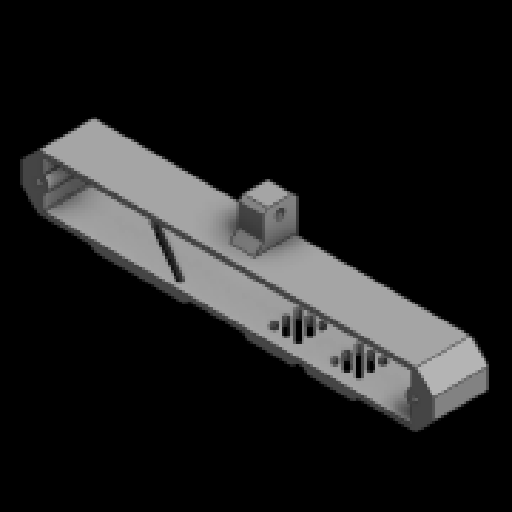
# Autodesk Inventor part: DepthCameraHousing
Saved by Autodesk Inventor 2025.2 (Build 292293000, 293)
## iProperties
Created: 2026-02-04
Part Number: DepthCameraHousing
Material: Generic
Document SubType Name: Modeling
Designer: valer
Density: 1 g/cm^3
Appearance: Default
Author: valer
Autodesk Inventor part; units mm, degrees
ref_plane "YZ Plane" through (0, 0, 0) normal (1, 0, 0) x (0, 1, 0)
ref_plane "XZ Plane" through (0, 0, 0) normal (0, 1, 0) x (-1, 0, 0)
ref_plane "XY Plane" through (0, 0, 0) normal (0, 0, 1) x (1, 0, 0)
sketch "Base" plane through (0, 0, 0) normal (0, 0, 1) x (1, 0, 0)
  line L0 (-81.75, 10.35) -> (81.75, 10.35)
  line L1 (81.75, 10.35) -> (81.75, -10.35)
  line L2 (81.75, -10.35) -> (-81.75, -10.35)
  line L3 (-81.75, -10.35) -> (-81.75, 10.35)
  line L4 (-81.75, 10.35) -> (81.75, -10.35) construction
  line L5 (81.75, 10.35) -> (-81.75, -10.35) construction
  line L6 (-122.5, 0) -> (122.5, 0) construction
  line L7 (0, -17.29) -> (0, 17.29) construction
  line L8 (83.75, 12.35) -> (-83.75, 12.35)
  line L9 (-83.75, 12.35) -> (-83.75, -12.35)
  line L10 (-83.75, -12.35) -> (83.75, -12.35)
  line L11 (83.75, -12.35) -> (83.75, 12.35)
  circle A0 centre (-83.5, 0) radius 4
  circle A1 centre (83.5, 0) radius 4
  line L12 (-83.5, 0) -> (83.5, 0) construction
  circle A2 centre (-83.5, 0) radius 1
  circle A3 centre (83.5, 0) radius 1
  point P0 (0, 0)
  point P1 (-83.75, 3.9922)
  point P2 (-83.75, -3.9922)
  point P3 (83.75, -3.9922)
  point P4 (83.75, 3.9922)
  point P5 (-81.75, 3.5969)
  point P6 (81.75, 3.5969)
  point P7 (81.75, -3.5969)
  point P8 (-81.75, -3.5969)
  dimension "d0" = 20.7
  dimension "d14" = 2
  dimension "d51" = 8
  dimension "d52" = 167
  dimension "d53" = 163.5
  dimension "d54" = 2
  dimension "d55" = 2
  constraints: 22 end point, 4 centre point, 4 parallel, 3 midpoint, 2 coincident, 2 perpendicular, 2 point on line, 1 collinear, 1 equal radius, 1 horizontal, 3 other
  measures "d0" distance between parallel lines of L2 L0
  measures "d14" distance between parallel lines of L0 L8
  measures "d51" diameter of A0
  measures "d52" distance of L12.end L12.start
  measures "d53" distance between parallel lines of L1 L3
  measures "d54" diameter of A2
  measures "d55" diameter of A3
extrude "BaseFeature" add sketch "Base" along normal blind 22.5 contours L3 A0 L9 L8 L11 A1 L1 L0 | A0 L3 | L3 A0 L9 A2 | A1 L11 A3 L1 | L1 A1 | L3 L2 L1 A1 L11 L10 L9 A0 | L9 A2 A0 | A1 L11 A3
extrude "BackFeature" add sketch "Base" against normal blind 3 contours L3 A0 L9 L8 L11 A1 L1 L0 | L0 L1 A1 L2 L3 A0 | A0 L3 | L3 A0 L9 A2 | A1 L11 A3 L1 | L1 A1 | L3 L2 L1 A1 L11 L10 L9 A0 | L9 A2 A0 | A1 L11 A3
sketch "Mount" plane through (0, 0, -3) normal (0, 0, -1) x (-1, 0, 0)
  line L0 (126, 0) -> (-126, 0) construction
  line L1 (0, -19.25) -> (0, 19.25) construction
  line L2 (83.75, 12.35) -> (-83.75, 12.35) projected
  line L3 (5.5, 12.35) -> (2.5, 12.35)
  line L4 (5.5, 28.35) -> (5.5, 12.35)
  line L5 (-5.5, 28.35) -> (-5.5, 12.35)
  line L6 (5.5, 28.35) -> (-5.5, 28.35)
  point P0 (0, 0)
  point P1 (-5.5, 12.35)
  dimension "d70" = 16
  dimension "d121" = 11
  constraints: 12 end point, 3 horizontal, 2 symmetric about line, 1 point on line, 1 vertical, 4 other
  measures "d70" distance of L4.start L3.start
  measures "d121" distance between parallel lines of L5 L4
extrude "MountFeature" add sketch "Mount" against normal blind 15
chamfer "MountChamferFeature" distance 2 angle 45 2 edges at (0, 28.35, -3) (0, 28.35, 12)
sketch "Sides" plane through (0, 0, -3) normal (0, 0, -1) x (-1, 0, 0)
  line L0 (0, -20.568) -> (0, 36.503) construction
  line L1 (-83.75, -12.35) -> (83.75, -12.35) projected
  line L2 (-83.75, -12.35) -> (-91.5, -4.6)
  line L3 (128.1, 0) -> (-128.1, 0) construction
  line L4 (-91.5, -4.6) -> (-91.5, 0)
  arc A0 (-77.585, 12.415) -> (-77.585, -12.415) centre (-77.585, 0) ccw construction
  arc A1 (-83.75, 3.9922) -> (-83.75, -3.9922) centre (-83.5, 0) ccw projected
  line L5 (83.75, -12.35) -> (91.5, -4.6)
  line L6 (91.5, -4.6) -> (91.5, 0)
  line L7 (-83.75, 12.35) -> (-91.5, 4.6)
  line L8 (-91.5, 4.6) -> (-91.5, 0)
  line L9 (83.75, 12.35) -> (91.5, 4.6)
  line L10 (91.5, 4.6) -> (91.5, 0)
  line L11 (83.75, -12.35) -> (83.75, -3.9922) projected
  arc A2 (83.75, -3.9922) -> (83.75, 3.9922) centre (83.5, 0) ccw projected
  line L12 (83.75, 3.9922) -> (83.75, 12.35) projected
  line L13 (-83.75, -3.9922) -> (-83.75, -12.35) projected
  line L14 (-83.75, 12.35) -> (-83.75, 3.9922) projected
  point P0 (0, 0)
  point P1 (-87.5, 0)
  dimension "d76" = 4
  dimension "d77" = 45
  constraints: 16 end point, 6 symmetric about line, 1 perpendicular, 1 point on circle, 1 point on line
  measures "d76" distance of L4.end point (-87.5, 0)
  measures "d77" angle of L2 L3
extrude "SidesFeature" add sketch "Sides" against normal up to surface (25.5 mm away)
sketch "Decorative" plane through (0, 0, 22.5) normal (0, 0, 1) x (1, 0, 0)
  line L0 (-83.75, -12.35) -> (83.75, -12.35) projected
  line L1 (58, -12.35) -> (56, -14.35)
  line L2 (56, -14.35) -> (36, -14.35)
  line L3 (36, -14.35) -> (34, -12.35)
  circle A0 centre (46, 0) radius 9.875 construction
  line L4 (46, -14.35) -> (46, 0) construction
  circle A1 centre (19, 0) radius 9.875 construction
  line L5 (31, -12.35) -> (29, -14.35)
  line L6 (29, -14.35) -> (9, -14.35)
  line L7 (9, -14.35) -> (7, -12.35)
  line L8 (19, -14.35) -> (19, 0) construction
  line L9 (-17, -12.35) -> (-19, -14.35)
  line L10 (-19, -14.35) -> (-59, -14.35)
  line L11 (-59, -14.35) -> (-61, -12.35)
  point P0 (0, 0)
  dimension "d80" = 45
  dimension "d81" = 45
  dimension "d82" = 2
  dimension "d83" = 20
  dimension "d84" = 45
  dimension "d85" = 45
  dimension "d86" = 40
  dimension "d89" = 45
  dimension "d90" = 45
  dimension "d91" = 24
  constraints: 22 end point, 6 point on line, 3 collinear, 2 midpoint, 2 perpendicular, 1 horizontal, 1 parallel, 1 vertical
  measures "d80" angle of L0 L3
  measures "d81" angle of L0 L1
  measures "d82" distance between parallel lines of L0 L2
  measures "d83" distance of L1.end L2.end
  measures "d84" angle of L0 L5
  measures "d85" angle of L0 L7
  measures "d86" distance of L9.end L10.end
  measures "d89" angle of L0 L9
  measures "d90" angle of L0 L11
  measures "d91" distance of L9.start L7.end
extrude "DecorativeFeature" add sketch "Decorative" against normal up to surface (25.5 mm away)
chamfer "BackChamferFeature" distance 1 angle 45 21 edges at (-72.375, -12.35, -3) (-87.625, -8.475, -3) (-91.5, 0, -3) (-87.625, 8.475, -3) (-44.625, 12.35, -3) (-60, -13.35, -3) (-39, -14.35, -3) (-18, -13.35, -3) (-5, -12.35, -3) (8, -13.35, -3) (19, -14.35, -3) (30, -13.35, -3) (32.5, -12.35, -3) (35, -13.35, -3) (46, -14.35, -3) (57, -13.35, -3) (70.875, -12.35, -3) (87.625, -8.475, -3) (91.5, 0, -3) (87.625, 8.475, -3) (44.625, 12.35, -3)
sketch "MountHole" plane through (5.5, 12.35, 12) normal (1, 0, 0) x (0, 0, -1)
  line L0 (13, 16) -> (2, 16) projected
  line L1 (7.5, 16) -> (7.5, 11) construction
  circle A0 centre (7.5, 11) radius 2
  point P0 (12, -12.35)
  point P1 (15, 16)
  point P2 (0, 16)
  dimension "d97" = 4
  dimension "d98" = 5
  constraints: 2 end point, 1 centre point, 1 coincident, 1 midpoint, 1 vertical
  measures "d97" diameter of A0
  measures "d98" distance of L1.start L1.end
extrude "MountHoleFeature" cut sketch "MountHole" along normal through all both and the other way through all
sketch "DecorativeHoles" plane through (36, -14.35, 22.5) normal (0, -1, 0) x (1, 0, 0)
  line L0 (20, -24.5) -> (0, -24.5) construction
  line L1 (20, 0) -> (20, -24.5) construction
  line L2 (0, 0) -> (20, 0) construction
  line L3 (0, 0) -> (0, -24.5) construction
  line L4 (-7, -24.5) -> (-27, -24.5) construction
  line L5 (-7, 0) -> (-7, -24.5) construction
  line L6 (-27, 0) -> (-7, 0) construction
  line L7 (-27, 0) -> (-27, -24.5) construction
  line L8 (-55, -24.5) -> (-95, -24.5) construction
  line L9 (-55, 0) -> (-55, -24.5) construction
  line L10 (-95, 0) -> (-55, 0) construction
  line L11 (-95, 0) -> (-95, -24.5) construction
  line L12 (16, -6.5) -> (4, -18.5) construction
  line L13 (15.1161, -5.6161) -> (3.1161, -17.6161)
  line L14 (4.8839, -19.3839) -> (16.8839, -7.3839)
  arc A0 (16.8839, -7.3839) -> (15.1161, -5.6161) centre (16, -6.5) ccw
  arc A1 (3.1161, -17.6161) -> (4.8839, -19.3839) centre (4, -18.5) ccw
  line L15 (20, -18.5) -> (0, -18.5) construction
  line L16 (20, -4) -> (0, -4) construction
  line L17 (14.5858, -18.5) -> (16, -17.0858) construction
  line L18 (13.7019, -17.6161) -> (15.1161, -16.2019)
  line L19 (16.8839, -17.9697) -> (15.4697, -19.3839)
  arc A2 (13.7019, -17.6161) -> (15.4697, -19.3839) centre (14.5858, -18.5) ccw
  arc A3 (16.8839, -17.9697) -> (15.1161, -16.2019) centre (16, -17.0858) ccw
  line L20 (4, -7.9142) -> (5.4142, -6.5) construction
  line L21 (4.8839, -8.7981) -> (6.2981, -7.3839)
  line L22 (4.5303, -5.6161) -> (3.1161, -7.0303)
  arc A4 (3.1161, -7.0303) -> (4.8839, -8.7981) centre (4, -7.9142) ccw
  arc A5 (6.2981, -7.3839) -> (4.5303, -5.6161) centre (5.4142, -6.5) ccw
  line L23 (9.2929, -18.5) -> (16, -11.7929) construction
  line L24 (10.1768, -19.3839) -> (16.8839, -12.6768)
  line L25 (15.1161, -10.909) -> (8.409, -17.6161)
  arc A6 (8.409, -17.6161) -> (10.1768, -19.3839) centre (9.2929, -18.5) ccw
  arc A7 (16.8839, -12.6768) -> (15.1161, -10.909) centre (16, -11.7929) ccw
  line L26 (4, -13.2071) -> (10.7071, -6.5) construction
  line L27 (3.1161, -12.3232) -> (9.8232, -5.6161)
  line L28 (11.591, -7.3839) -> (4.8839, -14.091)
  arc A8 (3.1161, -12.3232) -> (4.8839, -14.091) centre (4, -13.2071) ccw
  arc A9 (11.591, -7.3839) -> (9.8232, -5.6161) centre (10.7071, -6.5) ccw
  line L29 (20, -18.5) -> (0, -4) construction
  line L30 (-2, -24.5) -> (-5, -24.5) projected
  line L31 (-5, 0) -> (-2, 0) projected
  line L32 (-10.1161, -17.9697) -> (-11.5303, -19.3839)
  arc A10 (-13.2981, -17.6161) -> (-11.5303, -19.3839) centre (-12.4142, -18.5) ccw
  arc A11 (-10.1161, -17.9697) -> (-11.8839, -16.2019) centre (-11, -17.0858) ccw
  line L33 (-13.2981, -17.6161) -> (-11.8839, -16.2019)
  line L34 (-16.8232, -19.3839) -> (-10.1161, -12.6768)
  arc A12 (-18.591, -17.6161) -> (-16.8232, -19.3839) centre (-17.7071, -18.5) ccw
  line L35 (-11.8839, -10.909) -> (-18.591, -17.6161)
  arc A13 (-10.1161, -12.6768) -> (-11.8839, -10.909) centre (-11, -11.7929) ccw
  line L36 (-22.1161, -19.3839) -> (-10.1161, -7.3839)
  arc A14 (-10.1161, -7.3839) -> (-11.8839, -5.6161) centre (-11, -6.5) ccw
  line L37 (-11.8839, -5.6161) -> (-23.8839, -17.6161)
  arc A15 (-23.8839, -17.6161) -> (-22.1161, -19.3839) centre (-23, -18.5) ccw
  arc A16 (-23.8839, -12.3232) -> (-22.1161, -14.091) centre (-23, -13.2071) ccw
  line L38 (-15.409, -7.3839) -> (-22.1161, -14.091)
  line L39 (-23.8839, -12.3232) -> (-17.1768, -5.6161)
  arc A17 (-15.409, -7.3839) -> (-17.1768, -5.6161) centre (-16.2929, -6.5) ccw
  arc A18 (-20.7019, -7.3839) -> (-22.4697, -5.6161) centre (-21.5858, -6.5) ccw
  line L40 (-22.1161, -8.7981) -> (-20.7019, -7.3839)
  line L41 (-22.4697, -5.6161) -> (-23.8839, -7.0303)
  arc A19 (-23.8839, -7.0303) -> (-22.1161, -8.7981) centre (-23, -7.9142) ccw
  point P0 (-36, -22.5)
  point P1 (10, -12.5)
  point P2 (15.2929, -17.7929)
  point P3 (12.6464, -15.1464)
  point P4 (4.7071, -7.2071)
  dimension "d102" = 45
  dimension "d104" = 4
  dimension "d105" = 4
  dimension "d106" = 4
  dimension "d107" = 4
  dimension "d108" = 3.7426
  dimension "d109" = 3.7426
  dimension "d110" = 3.7426
  dimension "d111" = 3.7426
  dimension "d113" = 4
  dimension "d114" = 4
  dimension "d115" = 4
  dimension "d118" = 6
  dimension "d119" = 2
  dimension "d120" = 1.25
  dimension "d124" = 27
  constraints: 66 end point, 40 point on circle, 20 centre point, 12 symmetric about line, 12 tangent, 7 point on line, 5 parallel, 4 midpoint, 2 equal radius, 2 perpendicular, 1 horizontal, 54 other
  measures "d102" angle of L12 L1
  measures "d104" distance from line of L1 L12.start
  measures "d105" distance between parallel lines of L2 L16
  measures "d106" distance from line of L1 L17.end
  measures "d107" distance from line of L1 L23.end
  measures "d108" distance between parallel lines of L23 L17
  measures "d109" distance between parallel lines of L12 L23
  measures "d110" distance between parallel lines of L26 L12
  measures "d111" distance from line of point (4.707, -7.207) L26
  measures "d113" distance from line of L3 L20.start
  measures "d114" distance from line of L3 L12.end
  measures "d115" distance from line of L3 L26.start
  measures "d118" distance between parallel lines of L0 L15
  measures "d119" distance of L17.start L17.end
  measures "d120" radius of A1
  measures "d124" distance of L19.start L32.start
extrude "DecorativeHolesFeature" cut sketch "DecorativeHoles" against normal up to surface (4 mm away)
sketch "OneMoreDecorativeHole" plane through (-59, -14.35, 22.5) normal (0, -1, 0) x (1, 0, 0)
  line L0 (34, -4) -> (6, -20.5) construction
  line L1 (33.3654, -2.9231) -> (5.3654, -19.4231)
  line L2 (6.6346, -21.5769) -> (34.6346, -5.0769)
  arc A0 (34.6346, -5.0769) -> (33.3654, -2.9231) centre (34, -4) ccw
  arc A1 (5.3654, -19.4231) -> (6.6346, -21.5769) centre (6, -20.5) ccw
  arc A2 (71.1161, -17.6161) -> (72.8839, -19.3839) centre (72, -18.5) ccw projected
  line L3 (0, 0) -> (40, 0) projected
  line L4 (40, 0) -> (40, -24.5) projected
  line L5 (0, 0) -> (0, -24.5) projected
  line L6 (40, -24.5) -> (0, -24.5) projected
  point P0 (59, -22.5)
  point P1 (20, -12.25)
  dimension "d132" = 4
  dimension "d133" = 6
  dimension "d134" = 6
  dimension "d135" = 4
  constraints: 8 end point, 4 point on circle, 4 tangent, 2 centre point, 1 equal radius, 1 midpoint, 1 parallel
  measures "d132" distance from line of L3 L0.start
  measures "d133" distance from line of L4 L0.start
  measures "d134" distance from line of L5 L0.end
  measures "d135" distance from line of L6 L0.end
chamfer "FrontChamferFeature" distance 4 angle 45 1 edges at (0, 12.35, 12)
extrude "OneMoreDecorativeHoleFeature" cut sketch "OneMoreDecorativeHole" against normal up to surface (4 mm away) contours A0 L2 A1 L1
fillet "InsideFilletsFeature" radius 0.5 16 edges at (81.75, -10.35, 11.25) (81.75, -3.5969, 11.25) (81.75, 3.5969, 11.25) (81.75, 10.35, 11.25) (0, 10.35, 0) (81.75, 6.9734, 0) (79.5, 0, 0) (81.75, -6.9734, 0) (0, -10.35, 0) (-81.75, -6.9734, 0) (-79.5, 0, 0) (-81.75, -3.5969, 11.25) (-81.75, 3.5969, 11.25) (-81.75, 6.9734, 0) (-81.75, 10.35, 11.25) (-81.75, -10.35, 11.25)
equation "\"d81\" = d80"
equation "\"d84\" = d80"
equation "\"d89\" = d80"
equation "\"d90\" = d80"
equation "\"d104\" = d103"
equation "\"d105\" = d103"
equation "\"d106\" = d103"
equation "\"d107\" = d104"
equation "\"d109\" = d108"
equation "\"d110\" = d108"
equation "\"d111\" = d108"
equation "\"d103\" = 4"
body "Solid1"
